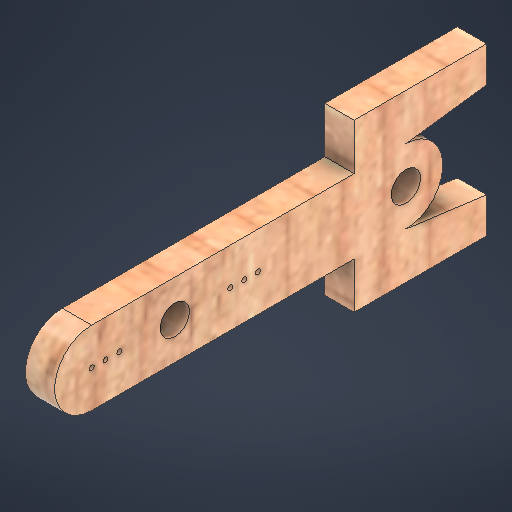
# Autodesk Inventor part: Crank Skiba
Saved by Autodesk Inventor 2026.2 (Build 302298000, 298)
## iProperties
Created: 2024-10-30
Part Number: Crank Skiba
Material: Generic
Document SubType Name: Modeling
Designer: 239tr
Density: 1 g/cm^3
Appearance: Birch - Natural Polished
Mass: 11.1341 g
Surface Area: 57.4576 cm^2
Volume: 11.1341 cm^3
Author: 239tr
Autodesk Inventor part; units mm, degrees
ref_plane "YZ Plane" through (0, 0, 0) normal (1, 0, 0) x (0, 1, 0)
ref_plane "XZ Plane" through (0, 0, 0) normal (0, 1, 0) x (-1, 0, 0)
ref_plane "XY Plane" through (0, 0, 0) normal (0, 0, 1) x (1, 0, 0)
sketch "Block1" plane through (0, 0, 0) normal (0, 0, 1) x (1, 0, 0)
  circle A0 centre (-34.5082, -40.3774) radius 0.55
  circle A1 centre (-31.5082, -40.3774) radius 0.55
  circle A2 centre (-28.5082, -40.3774) radius 0.55
  point P0 (-31.5082, -40.3774)
  dimension "d7" = 1.1
  dimension "d8" = 1.1
  dimension "d9" = 1.1
  measures "d7" diameter of A0
  measures "d8" diameter of A1
  measures "d9" diameter of A2
sketch "Sketch1" plane through (0, 0, 0) normal (1, 0, 0) x (0, 1, 0)
  circle A0 centre (0, 0) radius 3.175
  line L0 (8, 0) -> (8, -50)
  line L1 (-8, 0) -> (-8, -50)
  arc A1 (-8, -50) -> (8, -50) centre (0, -50) ccw
  circle A2 centre (0, -50) radius 3.175
  line L2 (0, -86.2) -> (0, 44.7) construction
  line L3 (8, 0) -> (-8, 0) construction
  line L4 (8, 0) -> (8, 18)
  line L5 (-8, 0) -> (-8, 18)
  arc A3 (8, 18) -> (-8, 18) centre (0, 18) ccw
  line L6 (-25.2, 0) -> (25.2, 0) construction
  line L7 (-8, -42.5) -> (-18, -42.5)
  line L8 (-18, -42.5) -> (-18, -67.5)
  line L9 (-18, -67.5) -> (-8, -67.5)
  line L10 (-8, -67.5) -> (-8, -42.5)
  line L11 (-8, -42.5) -> (17.0955, -42.5) construction
  line L12 (-8, -50) -> (-18, -50)
  line L13 (-18, -50) -> (-18, -38.8151)
  line L14 (-18, -38.8151) -> (-8, -38.8151)
  line L15 (-8, -38.8151) -> (-8, -50)
  line L16 (-8, -50) -> (-10.3039, -67.5)
  line L17 (-8, -50) -> (9.651, -50) construction
  line L18 (8, -42.5) -> (18, -42.5)
  line L19 (18, -42.5) -> (18, -67.5)
  line L20 (18, -67.5) -> (8, -67.5)
  line L21 (8, -67.5) -> (8, -42.5)
  line L22 (8, -50) -> (18, -50)
  line L23 (18, -50) -> (18, -38.8151)
  line L24 (18, -38.8151) -> (8, -38.8151)
  line L25 (8, -38.8151) -> (8, -50)
  line L26 (8, -50) -> (10.3039, -67.5)
  circle A4 centre (0, -12) radius 0.55
  circle A5 centre (0, -15) radius 0.55
  circle A6 centre (0, -18) radius 0.55
  circle A7 centre (0, 12) radius 0.55
  circle A8 centre (0, 15) radius 0.55
  circle A9 centre (0, 18) radius 0.55
  point P0 (0, 0)
  point P1 (-8, -25)
  dimension "d0" = 6.35
  dimension "d2" = 16
  dimension "d4" = 6.35
  dimension "d11" = 12
  dimension "d12" = 50
  dimension "d16" = 10
  dimension "d17" = 25
  dimension "d18" = 42.5
  dimension "d20" = 10
  dimension "d21" = 97.5
  constraints: 50 end point, 8 symmetric about line, 8 vertical, 5 horizontal, 4 centre point, 4 parallel, 4 point on circle, 4 tangent, 3 point on line, 2 coincident, 2 midpoint, 2 perpendicular, 1 collinear, 1 equal length, 1 other
  measures "d0" diameter of A0
  measures "d2" diameter of A1
  measures "d4" diameter of A2
  measures "d12" distance of A1.centre A0.centre
  measures "d16" distance of L9.end L8.end
  measures "d17" distance of L8.end L7.end
  measures "d18" distance between parallel lines of L7 L6
  measures "d20" distance of L13.end L14.end
  measures "d21" angle of L16 L17
extrude "Extrusion1" add sketch "Sketch1" along normal blind 6.35 contours L0 A1 L1 L5 A3 L4 | L24 L23 L18 L0 | L18 L19 L22 L0 | L22 L19 L20 L26 | L12 L8 L7 L1 | L16 L9 L8 L12 | L1 L7 L13 L14
equation "\"d7\" = d9"
equation "\"d8\" = d9"
body "Solid1"
